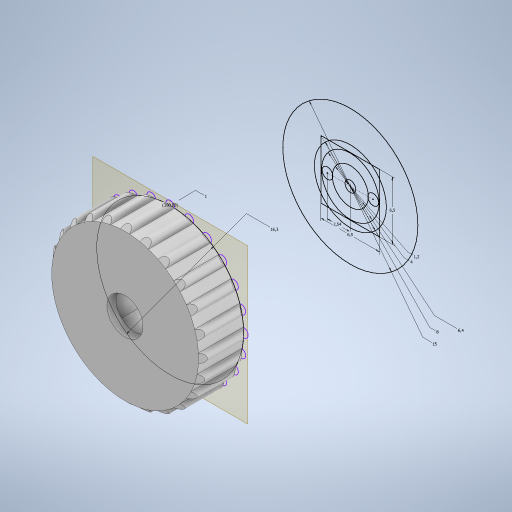
# Autodesk Inventor part: ATU_BUTN
Saved by Autodesk Inventor 2024 (Build 280153000, 153)
## iProperties
Created: 2024-11-27
Part Number: ATU_BUTN
Material: Типовые
Document SubType Name: Modeling
Designer: fm
Density: 1 g/cm^3
Appearance: По умолчанию
Author: fm
Autodesk Inventor part; units mm, degrees
ref_plane "YZ Plane" through (0, 0, 0) normal (1, 0, 0) x (0, 1, 0)
ref_plane "XZ Plane" through (0, 0, 0) normal (0, 1, 0) x (-1, 0, 0)
ref_plane "XY Plane" through (0, 0, 0) normal (0, 0, 1) x (1, 0, 0)
sketch "Эскиз1" plane through (0, 0, 0) normal (0, 0, 1) x (1, 0, 0)
  circle A0 centre (0, 0) radius 3.2
  circle A1 centre (0, 0) radius 7.5
  circle A2 centre (0, 0) radius 0.6
  circle A3 centre (2.54, 0) radius 0.6
  circle A4 centre (-2.54, 0) radius 0.6
  circle A5 centre (0, 0) radius 4
  line L0 (-2.54, 0) -> (2.54, 0) construction
  circle A6 centre (0, 0) radius 2
  line L1 (-3.25, 3.25) -> (3.25, 3.25)
  line L2 (3.25, 3.25) -> (3.25, -3.25)
  line L3 (3.25, -3.25) -> (-3.25, -3.25)
  line L4 (-3.25, -3.25) -> (-3.25, 3.25)
  line L5 (-3.25, 3.25) -> (3.25, -3.25) construction
  point P0 (3.088898, 0.83589)
  point P1 (-3.088898, 0.83589)
  point P2 (-3.088898, -0.83589)
  point P3 (3.088898, -0.83589)
  dimension "d0" = 6.4
  dimension "d1" = 15
  dimension "d2" = 1.2
  dimension "d7" = 8
  dimension "d9" = 2.54
  dimension "d10" = 4
  dimension "d33" = 6.5
  dimension "d34" = 6.5
  constraints: 12 end point, 8 coincident, 7 centre point, 2 equal radius, 2 horizontal, 2 midpoint, 2 parallel, 1 perpendicular
  measures "d0" diameter of A0
  measures "d1" diameter of A1
  measures "d2" diameter of A2
  measures "d7" diameter of A5
  measures "d9" distance of point (0, 0) L0.start
  measures "d10" diameter of A6
  measures "d33" distance of L2.end L3.end
  measures "d34" distance of L1.end L2.end
extrude "Выдавливание1" add sketch "Эскиз1" against normal blind 2 contours A0 | A1 | A2 | A3 A6 A4 | A5 L2 | L2 A5 L3 L4 L1 | A5 L1 L2 | L2 L3 A5 | L1 A5 | A5 L3 | A5 L4 L1 | L3 L4 A5 | L4 A5
chamfer "Фаска1" distance 0.5 angle 45 1 edges at (-7.5, 0, -2)
ref_plane "РабПлоскость1" through (0, 0, 20) normal (0, 0, 1) x (1, 0, 0)
sketch "Эскиз2" plane through (0, 0, 20) normal (0, 0, 1) x (1, 0, 0)
  circle A0 centre (0, 0) radius 8.15
  circle A1 centre (0, 8.15) radius 0.5
  circle A2 centre (0, 0) radius 2
  circle A3 centre (-2.109375, 7.872295) radius 0.5
  circle A4 centre (-4.075, 7.058107) radius 0.5
  circle A5 centre (-5.76292, 5.76292) radius 0.5
  circle A6 centre (-7.058107, 4.075) radius 0.5
  circle A7 centre (-7.872295, 2.109375) radius 0.5
  circle A8 centre (-8.15, 0) radius 0.5
  circle A9 centre (-7.872295, -2.109375) radius 0.5
  circle A10 centre (-7.058107, -4.075) radius 0.5
  circle A11 centre (-5.76292, -5.76292) radius 0.5
  circle A12 centre (-4.075, -7.058107) radius 0.5
  circle A13 centre (-2.109375, -7.872295) radius 0.5
  circle A14 centre (0, -8.15) radius 0.5
  circle A15 centre (2.109375, -7.872295) radius 0.5
  circle A16 centre (4.075, -7.058107) radius 0.5
  circle A17 centre (5.76292, -5.76292) radius 0.5
  circle A18 centre (7.058107, -4.075) radius 0.5
  circle A19 centre (7.872295, -2.109375) radius 0.5
  circle A20 centre (8.15, 0) radius 0.5
  circle A21 centre (7.872295, 2.109375) radius 0.5
  circle A22 centre (7.058107, 4.075) radius 0.5
  circle A23 centre (5.76292, 5.76292) radius 0.5
  circle A24 centre (4.075, 7.058107) radius 0.5
  circle A25 centre (2.109375, 7.872295) radius 0.5
  point P0 (5.398688, 6.105462)
  point P1 (6.105462, 5.398688)
  point P2 (3.634522, 7.294707)
  point P3 (4.50014, 6.794942)
  point P4 (1.62267, 7.986829)
  point P5 (2.588141, 7.728132)
  point P6 (0.499765, 8.134663)
  point P7 (-0.499765, 8.134663)
  point P8 (-2.588141, 7.728132)
  point P9 (-1.62267, 7.986829)
  point P10 (-4.50014, 6.794942)
  point P11 (-3.634522, 7.294707)
  point P12 (-6.105462, 5.398688)
  point P13 (-5.398688, 6.105462)
  point P14 (-7.294707, 3.634522)
  point P15 (-6.794942, 4.50014)
  point P16 (-7.986829, 1.62267)
  point P17 (-7.728132, 2.588141)
  point P18 (-8.134663, -0.499765)
  point P19 (-8.134663, 0.499765)
  point P20 (-7.728132, -2.588141)
  point P21 (-7.986829, -1.62267)
  point P22 (-6.794942, -4.50014)
  point P23 (-7.294707, -3.634522)
  point P24 (-5.398688, -6.105462)
  point P25 (-6.105462, -5.398688)
  point P26 (-3.634522, -7.294707)
  point P27 (-4.50014, -6.794942)
  point P28 (-1.62267, -7.986829)
  point P29 (-2.588141, -7.728132)
  point P30 (-0.499765, -8.134663)
  point P31 (0.499765, -8.134663)
  point P32 (2.588141, -7.728132)
  point P33 (1.62267, -7.986829)
  point P34 (4.50014, -6.794942)
  point P35 (3.634522, -7.294707)
  point P36 (6.105462, -5.398688)
  point P37 (5.398688, -6.105462)
  point P38 (7.294707, -3.634522)
  point P39 (6.794942, -4.50014)
  point P40 (7.986829, -1.62267)
  point P41 (7.728132, -2.588141)
  point P42 (8.134663, 0.499765)
  point P43 (8.134663, -0.499765)
  point P44 (7.728132, 2.588141)
  point P45 (7.986829, 1.62267)
  point P46 (6.794942, 4.50014)
  point P47 (7.294707, 3.634522)
  dimension "d23" = 16.3
  dimension "d35" = 1
  dimension "d38" = 360
  constraints: 24 centre point, 1 coincident, 52 other
  measures "d35" diameter of A1
extrude "Выдавливание5" add sketch "Эскиз2" along normal blind 5 separate body contours A0 A20 | A0 A20 | A20 A0 A19 A18 A17 A16 A15 A14 A13 A12 A11 A10 A9 A8 A7 A6 A5 A4 A3 A1 A25 A24 A23 A22 A21 | A21 A0 | A0 A21 | A19 A0 | A0 A19 | A22 A0 | A0 A22 | A18 A0 | A0 A18 | A23 A0 | A0 A23 | A17 A0 | A0 A17 | A24 A0 | A0 A24 | A16 A0 | A0 A16 | A25 A0 | A0 A25 | A15 A0 | A0 A15 | A1 A0 | A0 A1 | A14 A0 | A0 A14 | A3 A0 | A0 A3 | A13 A0 | A0 A13 | A4 A0 | A0 A4 | A12 A0 | A0 A12 | A5 A0 | A0 A5 | A11 A0 | A0 A11 | A6 A0 | A0 A6 | A10 A0 | A0 A10 | A7 A0 | A0 A7 | A9 A0 | A0 A9 | A8 A0 | A0 A8 | A2
extrude "Выдавливание6" cut sketch "Эскиз1" along normal up to surface (5 mm away) from surface at 20 contours A2 | A6 A3 | A3 A6 A4 | A4 A6 picked at (1.963417, -0.065179) picked at (-1.979002, 0) bodies 2
extrude "Выдавливание7" cut sketch "Эскиз1" along normal blind 4 from surface at 20 contours A0 | A2 | A3 A6 | A6 A3 | A3 A6 A4 | A6 A4 | A4 A6 | L2 A5 L3 L4 L1 | A5 L1 L2 | L2 L3 A5 | A5 L4 L1 | L3 L4 A5 bodies 2
sketch "Эскиз3" plane through (0, 0, 0) normal (1, 0, 0) x (0, 1, 0)
  line L0 (8.65, 20) -> (8.65, 25) projected
  line L1 (8.65, 25) -> (8.15, 25)
  line L2 (8.15, 25) -> (8.65, 24.5)
  line L3 (8.65, 20) -> (8.15, 20)
  line L4 (8.15, 20) -> (8.65, 20.5)
  line L5 (0, -5) -> (0, 30) projected
  point P0 (0, 0)
  dimension "d40" = 0.5
  dimension "d42" = 45
  dimension "d43" = 0.5
  dimension "d45" = 45
  constraints: 8 end point, 2 horizontal, 2 point on line
  measures "d40" distance of L0.end L1.end
  measures "d42" angle of L2 L1
  measures "d43" distance of L0.start L3.end
  measures "d45" angle of L3 L4
revolve "Вращение1" cut sketch "Эскиз3" angle 360 about axis through (0, 0, -10) along (0, 0, 1) bodies 2
